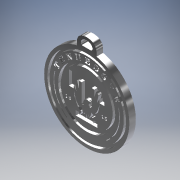
# Autodesk Inventor part: Aluminum Backing
Saved by Autodesk Inventor 2018 (Build 220112000, 112)
## iProperties
Created: 2017-11-28
Part Number: Aluminum Backing
Material: Aluminum 6061
Document SubType Name: Modeling
Designer: Rus
Density: 2.7 g/cm^3
Appearance: Aluminum - Flat
Author: Rus
Autodesk Inventor part; units mm, degrees
(part 1 of 2)
ref_plane "YZ Plane" through (0, 0, 0) normal (1, 0, 0) x (0, 1, 0)
ref_plane "XZ Plane" through (0, 0, 0) normal (0, 1, 0) x (-1, 0, 0)
ref_plane "XY Plane" through (0, 0, 0) normal (0, 0, 1) x (1, 0, 0)
sketch "Sketch1" plane through (0, 0, 0) normal (0, 0, 1) x (1, 0, 0)
  circle A0 centre (0, 0) radius 41.275
  line L0 (-9.525, 40.1609) -> (-9.525, 43.3359)
  line L1 (9.525, 43.3359) -> (9.525, 40.1609)
  line L2 (-9.525, 43.3359) -> (-9.525, 52.8609) construction
  line L3 (-9.525, 52.8609) -> (0, 52.8609) construction
  line L4 (0, 52.8609) -> (9.525, 52.8609) construction
  line L5 (9.525, 52.8609) -> (9.525, 43.3359) construction
  spline S0 degree 4 poles (-9.525, 43.3359) (-9.525, 52.8609) (0, 52.8609) (9.525, 52.8609) (9.525, 43.3359) knots 1 1 1 1 1 2 2 2 2 2
  line L6 (0, 0) -> (0, 52.8609) construction
  line L7 (-9.525, 40.1609) -> (-9.525, 52.8609) construction
  line L8 (-3.7012, 44.5588) -> (3.7012, 44.5588) construction
  line L9 (3.7012, 42.545) -> (-3.7012, 42.545)
  arc A1 (-5.715, 44.5588) -> (-3.7012, 42.545) centre (-3.7012, 44.5588) ccw
  arc A2 (3.7012, 42.545) -> (5.715, 44.5588) centre (3.7012, 44.5588) ccw
  line L10 (-5.715, 44.5588) -> (-5.715, 48.3682) construction
  line L11 (-5.715, 48.3682) -> (0, 51.6703) construction
  line L12 (0, 51.6703) -> (5.715, 48.3682) construction
  line L13 (5.715, 48.3682) -> (5.715, 44.5588) construction
  spline S1 degree 4 poles (-5.715, 44.5588) (-5.715, 48.3682) (0, 51.6703) (5.715, 48.3682) (5.715, 44.5588) knots 0 0 0 0 0 1 1 1 1 1
  point P0 (0, 44.5588)
  point P1 (0, 41.275)
  point P2 (0, 49.1303)
  dimension "d0" = 82.55
  dimension "d1" = 9.525
  dimension "d2" = 12.7
  dimension "d3" = 1.27
  dimension "d4" = 19.05
  dimension "d5" = 3.81
  dimension "d6" = 2.54
  constraints: 14 end point, 7 point on circle, 5 equal length, 5 vertical, 4 point on line, 3 centre point, 3 coincident, 3 horizontal, 2 tangent, 1 collinear, 1 midpoint, 1 parallel, 1 perpendicular, 10 other
  measures "d0" diameter of A0
  measures "d1" distance of L0.end L2.end
  measures "d2" distance of L2.end L0.start
  measures "d3" distance from line of L9 point (0, 41.275)
  measures "d4" distance between parallel lines of L5 L7
  measures "d5" distance from line of L2 L10.start
  measures "d6" distance of L11.end point (0, 49.13)
extrude "Extrusion1" add sketch "Sketch1" against normal blind 6.35
sketch "Sketch2" plane through (0, 0, 0) normal (0, 0, 1) x (1, 0, 0)
  line L0 (-17.3416, 16.1127) -> (17.1721, 16.1127) projected
  line L1 (-17.3416, 2.4226) -> (-17.3416, 16.1127) projected
  line L2 (-12.5842, 2.4226) -> (-17.3416, 2.4226) projected
  line L3 (-12.5842, 2.8144) -> (-12.5842, 2.4226) projected
  line L4 (-12.5284, 3.9883) -> (-12.5842, 2.8144) projected
  line L5 (-12.3951, 5.1768) -> (-12.5284, 3.9883) projected
  line L6 (-12.3568, 5.3992) -> (-12.3951, 5.1768) projected
  line L7 (-10.0045, 1.3116) -> (-12.3568, 5.3992) projected
  line L8 (-11.6489, 8.1267) -> (-10.0045, 1.3116) projected
  line L9 (-11.523, 8.419) -> (-11.6489, 8.1267) projected
  line L10 (-10.7114, 9.6284) -> (-11.523, 8.419) projected
  line L11 (-9.6469, 10.5162) -> (-10.7114, 9.6284) projected
  line L12 (-9.3949, 10.6484) -> (-9.6469, 10.5162) projected
  line L13 (-7.5644, 4.9816) -> (-9.3949, 10.6484) projected
  line L14 (-7.4901, 11.2654) -> (-7.5644, 4.9816) projected
  line L15 (-7.3021, 11.2986) -> (-7.4901, 11.2654) projected
  line L16 (-6.2911, 11.3978) -> (-7.3021, 11.2986) projected
  line L17 (-5.1831, 11.4155) -> (-6.2911, 11.3978) projected
  line L18 (-4.9463, 11.4069) -> (-5.1831, 11.4155) projected
  line L19 (-4.9566, -5.366) -> (-4.9463, 11.4069) projected
  line L20 (-4.9566, -5.5437) -> (-4.9566, -5.366) projected
  line L21 (-4.8688, -6.0783) -> (-4.9566, -5.5437) projected
  line L22 (-4.6042, -6.6704) -> (-4.8688, -6.0783) projected
  line L23 (-4.1619, -7.031) -> (-4.6042, -6.6704) projected
  line L24 (-3.6867, -7.0879) -> (-4.1619, -7.031) projected
  line L25 (-3.5431, -7.0506) -> (-3.6867, -7.0879) projected
  line L26 (-3.4581, -7.0279) -> (-3.5431, -7.0506) projected
  line L27 (-3.2038, -6.7852) -> (-3.4581, -7.0279) projected
  line L28 (-3.1821, -6.3109) -> (-3.2038, -6.7852) projected
  line L29 (-3.2134, -6.1722) -> (-3.1821, -6.3109) projected
  line L30 (-3.2876, -5.8436) -> (-3.2134, -6.1722) projected
  line L31 (-3.3446, -4.8204) -> (-3.2876, -5.8436) projected
  line L32 (-3.148, -3.5625) -> (-3.3446, -4.8204) projected
  line L33 (-2.6706, -2.4546) -> (-3.148, -3.5625) projected
  line L34 (-1.9595, -1.5554) -> (-2.6706, -2.4546) projected
  line L35 (-1.0615, -0.9207) -> (-1.9595, -1.5554) projected
  line L36 (-0.0227, -0.6088) -> (-1.0615, -0.9207) projected
  line L37 (1.1099, -0.6761) -> (-0.0227, -0.6088) projected
  line L38 (2.0206, -1.0117) -> (1.1099, -0.6761) projected
  line L39 (2.2892, -1.1792) -> (2.0206, -1.0117) projected
  line L40 (2.462, -1.1853) -> (2.2892, -1.1792) projected
  line L41 (2.9787, -1.2796) -> (2.462, -1.1853) projected
  line L42 (3.4976, -1.5627) -> (2.9787, -1.2796) projected
  line L43 (3.7921, -2.0846) -> (3.4976, -1.5627) projected
  line L44 (3.8374, -2.7026) -> (3.7921, -2.0846) projected
  line L45 (3.8094, -2.9032) -> (3.8374, -2.7026) projected
  line L46 (3.3827, -2.6573) -> (3.8094, -2.9032) projected
  line L47 (2.5963, -2.8059) -> (3.3827, -2.6573) projected
  line L48 (2.4277, -2.9343) -> (2.5963, -2.8059) projected
  line L49 (2.0515, -3.4873) -> (2.4277, -2.9343) projected
  line L50 (1.9037, -4.2725) -> (2.0515, -3.4873) projected
  line L51 (2.0982, -5.0136) -> (1.9037, -4.2725) projected
  line L52 (2.4329, -5.4662) -> (2.0982, -5.0136) projected
  line L53 (2.5798, -5.5645) -> (2.4329, -5.4662) projected
  line L54 (2.7369, -5.6689) -> (2.5798, -5.5645) projected
  line L55 (3.3322, -5.8013) -> (2.7369, -5.6689) projected
  line L56 (4.0224, -5.5719) -> (3.3322, -5.8013) projected
  line L57 (4.5289, -4.9538) -> (4.0224, -5.5719) projected
  line L58 (4.7252, -4.2592) -> (4.5289, -4.9538) projected
  line L59 (4.7252, -4.0289) -> (4.7252, -4.2592) projected
  line L60 (4.7149, 11.4069) -> (4.7252, -4.0289) projected
  line L61 (4.9505, 11.4155) -> (4.7149, 11.4069) projected
  line L62 (6.0585, 11.3978) -> (4.9505, 11.4155) projected
  line L63 (7.0704, 11.2995) -> (6.0585, 11.3978) projected
  line L64 (7.2586, 11.2666) -> (7.0704, 11.2995) projected
  line L65 (7.3329, 4.9816) -> (7.2586, 11.2666) projected
  line L66 (9.1632, 10.6484) -> (7.3329, 4.9816) projected
  line L67 (9.4155, 10.5162) -> (9.1632, 10.6484) projected
  line L68 (10.4798, 9.6284) -> (9.4155, 10.5162) projected
  line L69 (11.2925, 8.4201) -> (10.4798, 9.6284) projected
  line L70 (11.4184, 8.1277) -> (11.2925, 8.4201) projected
  line L71 (9.7732, 1.3116) -> (11.4184, 8.1277) projected
  line L72 (12.1377, 5.4186) -> (9.7732, 1.3116) projected
  line L73 (12.175, 5.1957) -> (12.1377, 5.4186) projected
  line L74 (12.3063, 3.9997) -> (12.175, 5.1957) projected
  line L75 (12.3633, 2.8173) -> (12.3063, 3.9997) projected
  line L76 (12.3633, 2.4226) -> (12.3633, 2.8173) projected
  line L77 (17.1721, 2.4226) -> (12.3633, 2.4226) projected
  line L78 (17.1721, 16.1127) -> (17.1721, 2.4226) projected
  line L79 (2.2407, -15.384) -> (1.4356, -12.0529) projected
  line L80 (2.1269, -15.5143) -> (2.2407, -15.384) projected
  line L81 (1.5349, -16.0249) -> (2.1269, -15.5143) projected
  line L82 (0.9115, -16.3567) -> (1.5349, -16.0249) projected
  line L83 (0.7833, -16.399) -> (0.9115, -16.3567) projected
  line L84 (-0.0278, -12.3673) -> (0.7833, -16.399) projected
  line L85 (-0.7586, -16.4651) -> (-0.0278, -12.3673) projected
  line L86 (-0.9001, -16.4331) -> (-0.7586, -16.4651) projected
  line L87 (-1.5844, -16.1344) -> (-0.9001, -16.4331) projected
  line L88 (-2.2344, -15.6353) -> (-1.5844, -16.1344) projected
  line L89 (-2.3574, -15.5029) -> (-2.2344, -15.6353) projected
  line L90 (-1.5234, -12.0529) -> (-2.3574, -15.5029) projected
  line L91 (-3.1295, -14.4178) -> (-1.5234, -12.0529) projected
  line L92 (-3.2276, -14.241) -> (-3.1295, -14.4178) projected
  line L93 (-3.6814, -13.2064) -> (-3.2276, -14.241) projected
  line L94 (-4.0826, -11.9569) -> (-3.6814, -13.2064) projected
  line L95 (-4.1537, -11.6736) -> (-4.0826, -11.9569) projected
  line L96 (-4.9589, -9.0011) -> (-4.1537, -11.6736) projected
  line L97 (-5.0075, -9.1787) -> (-4.9589, -9.0011) projected
  line L98 (-5.2597, -9.6833) -> (-5.0075, -9.1787) projected
  line L99 (-5.67, -10.0624) -> (-5.2597, -9.6833) projected
  line L100 (-6.1547, -10.1876) -> (-5.67, -10.0624) projected
  line L101 (-6.6785, -10.11) -> (-6.1547, -10.1876) projected
  line L102 (-7.2057, -9.8774) -> (-6.6785, -10.11) projected
  line L103 (-7.7029, -9.5406) -> (-7.2057, -9.8774) projected
  line L104 (-8.1328, -9.1499) -> (-7.7029, -9.5406) projected
  line L105 (-8.387, -8.8583) -> (-8.1328, -9.1499) projected
  line L106 (-8.4595, -8.754) -> (-8.387, -8.8583) projected
  line L107 (-8.9215, -8.0882) -> (-8.4595, -8.754) projected
  line L108 (-10.1171, -5.9602) -> (-8.9215, -8.0882) projected
  line L109 (-11.3266, -3.1398) -> (-10.1171, -5.9602) projected
  line L110 (-12.1027, -0.4743) -> (-11.3266, -3.1398) projected
  line L111 (-12.4168, 1.2691) -> (-12.1027, -0.4743) projected
  line L112 (-12.4591, 1.8541) -> (-12.4168, 1.2691) projected
  line L113 (-12.4654, 1.7457) -> (-12.4591, 1.8541) projected
  line L114 (-12.4901, 0.5995) -> (-12.4654, 1.7457) projected
  line L115 (-12.4892, 0.4787) -> (-12.4901, 0.5995) projected
  line L116 (-12.4871, -0.1156) -> (-12.4892, 0.4787) projected
  line L117 (-12.2411, -1.9016) -> (-12.4871, -0.1156) projected
  line L118 (-11.499, -4.7419) -> (-12.2411, -1.9016) projected
  line L119 (-10.2455, -7.8052) -> (-11.499, -4.7419) projected
  line L120 (-8.9617, -10.1317) -> (-10.2455, -7.8052) projected
  line L121 (-8.4595, -10.856) -> (-8.9617, -10.1317) projected
  line L122 (-8.3923, -10.9532) -> (-8.4595, -10.856) projected
  line L123 (-8.1772, -11.2366) -> (-8.3923, -10.9532) projected
  line L124 (-7.8021, -11.6914) -> (-8.1772, -11.2366) projected
  line L125 (-7.3586, -12.1678) -> (-7.8021, -11.6914) projected
  line L126 (-6.875, -12.6141) -> (-7.3586, -12.1678) projected
  line L127 (-6.3777, -12.9822) -> (-6.875, -12.6141) projected
  line L128 (-5.8924, -13.2178) -> (-6.3777, -12.9822) projected
  line L129 (-5.4435, -13.2725) -> (-5.8924, -13.2178) projected
  line L130 (-5.1345, -13.162) -> (-5.4435, -13.2725) projected
  line L131 (-5.0601, -13.0948) -> (-5.1345, -13.162) projected
  line L132 (-5.0715, -13.1744) -> (-5.0601, -13.0948) projected
  line L133 (-5.3464, -13.9556) -> (-5.0715, -13.1744) projected
  line L134 (-5.3837, -14.0301) -> (-5.3464, -13.9556) projected
  line L135 (-6.9908, -17.1772) -> (-5.3837, -14.0301) projected
  line L136 (-6.9908, -14.5934) -> (-6.9908, -17.1772) projected
  line L137 (-7.0517, -14.6028) -> (-6.9908, -14.5934) projected
  line L138 (-7.7059, -14.6855) -> (-7.0517, -14.6028) projected
  line L139 (-7.7753, -14.6927) -> (-7.7059, -14.6855) projected
  line L140 (-7.9759, -14.7123) -> (-7.7753, -14.6927) projected
  line L141 (-9.0897, -14.7794) -> (-7.9759, -14.7123) projected
  line L142 (-10.2443, -14.8074) -> (-9.0897, -14.7794) projected
  line L143 (-10.6288, -14.8074) -> (-10.2443, -14.8074) projected
  line L144 (-10.6288, -19.3528) -> (-10.6288, -14.8074) projected
  line L145 (10.4076, -19.3528) -> (-10.6288, -19.3528) projected
  line L146 (10.4076, -14.8074) -> (10.4076, -19.3528) projected
  line L147 (10.015, -14.798) -> (10.4076, -14.8074) projected
  line L148 (8.4108, -14.7401) -> (10.015, -14.798) projected
  line L149 (7.2843, -14.6658) -> (8.4108, -14.7401) projected
  line L150 (7.1302, -14.6481) -> (7.2843, -14.6658) projected
  line L151 (7.1015, -14.6451) -> (7.1302, -14.6481) projected
  line L152 (6.8296, -14.6131) -> (7.1015, -14.6451) projected
  line L153 (6.8037, -14.61) -> (6.8296, -14.6131) projected
  line L154 (6.8037, -17.1772) -> (6.8037, -14.61) projected
  line L155 (5.1448, -13.9278) -> (6.8037, -17.1772) projected
  line L156 (5.1107, -13.8617) -> (5.1448, -13.9278) projected
  line L157 (4.9103, -13.2272) -> (5.1107, -13.8617) projected
  line L158 (4.9, -13.1517) -> (4.9103, -13.2272) projected
  line L159 (4.9783, -13.2076) -> (4.9, -13.1517) projected
  line L160 (5.2875, -13.2788) -> (4.9783, -13.2076) projected
  line L161 (5.732, -13.1931) -> (5.2875, -13.2788) projected
  line L162 (6.2084, -12.9418) -> (5.732, -13.1931) projected
  line L163 (6.6932, -12.5728) -> (6.2084, -12.9418) projected
  line L164 (7.1622, -12.1316) -> (6.6932, -12.5728) projected
  line L165 (7.5903, -11.6676) -> (7.1622, -12.1316) projected
  line L166 (7.9541, -11.2264) -> (7.5903, -11.6676) projected
  line L167 (8.1629, -10.9503) -> (7.9541, -11.2264) projected
  line L168 (8.229, -10.856) -> (8.1629, -10.9503) projected
  line L169 (8.7312, -10.1317) -> (8.229, -10.856) projected
  line L170 (10.014, -7.8052) -> (8.7312, -10.1317) projected
  line L171 (11.2675, -4.7419) -> (10.014, -7.8052) projected
  line L172 (12.0085, -1.9016) -> (11.2675, -4.7419) projected
  line L173 (12.2554, -0.1156) -> (12.0085, -1.9016) projected
  line L174 (12.2575, 0.4787) -> (12.2554, -0.1156) projected
  line L175 (12.2575, 0.5995) -> (12.2575, 0.4787) projected
  line L176 (12.2337, 1.7457) -> (12.2575, 0.5995) projected
  line L177 (12.2288, 1.8541) -> (12.2337, 1.7457) projected
  line L178 (12.1865, 1.2691) -> (12.2288, 1.8541) projected
  line L179 (11.871, -0.4743) -> (12.1865, 1.2691) projected
  line L180 (11.0951, -3.1398) -> (11.871, -0.4743) projected
  line L181 (9.8856, -5.9602) -> (11.0951, -3.1398) projected
  line L182 (8.69, -8.0882) -> (9.8856, -5.9602) projected
  line L183 (8.229, -8.754) -> (8.69, -8.0882) projected
  line L184 (8.1555, -8.8583) -> (8.229, -8.754) projected
  line L185 (7.9002, -9.1499) -> (8.1555, -8.8583) projected
  line L186 (7.4703, -9.5406) -> (7.9002, -9.1499) projected
  line L187 (6.9742, -9.8774) -> (7.4703, -9.5406) projected
  line L188 (6.4461, -10.11) -> (6.9742, -9.8774) projected
  line L189 (5.9221, -10.1876) -> (6.4461, -10.11) projected
  line L190 (5.4374, -10.0624) -> (5.9221, -10.1876) projected
  line L191 (5.0281, -9.6833) -> (5.4374, -10.0624) projected
  line L192 (4.777, -9.1775) -> (5.0281, -9.6833) projected
  line L193 (4.7284, -9.0011) -> (4.777, -9.1775) projected
  line L194 (3.9232, -11.6736) -> (4.7284, -9.0011) projected
  line L195 (3.855, -11.9424) -> (3.9232, -11.6736) projected
  line L196 (3.478, -13.134) -> (3.855, -11.9424) projected
  line L197 (3.0541, -14.1315) -> (3.478, -13.134) projected
  line L198 (2.963, -14.3041) -> (3.0541, -14.1315) projected
  line L199 (1.4356, -12.0529) -> (2.963, -14.3041) projected
  line L200 (-15.909, -6.753) -> (-16.0207, -6.4378) projected
  line L201 (-15.909, -6.9639) -> (-15.909, -6.753) projected
  line L202 (-16.0176, -7.2586) -> (-15.909, -6.9639) projected
  line L203 (-16.0393, -7.2841) -> (-16.0176, -7.2586) projected
  line L204 (-16.0611, -7.3102) -> (-16.0393, -7.2841) projected
  line L205 (-16.3039, -7.4392) -> (-16.0611, -7.3102) projected
  line L206 (-16.488, -7.4392) -> (-16.3039, -7.4392) projected
  line L207 (-16.7731, -7.3112) -> (-16.488, -7.4392) projected
  line L208 (-16.7958, -7.2864) -> (-16.7731, -7.3112) projected
  line L209 (-16.8196, -7.2605) -> (-16.7958, -7.2864) projected
  line L210 (-16.9364, -6.9513) -> (-16.8196, -7.2605) projected
  line L211 (-16.9364, -6.7376) -> (-16.9364, -6.9513) projected
  line L212 (-16.828, -6.4296) -> (-16.9364, -6.7376) projected
  line L213 (-16.8051, -6.4048) -> (-16.828, -6.4296) projected
  line L214 (-16.7834, -6.3789) -> (-16.8051, -6.4048) projected
  line L215 (-16.5209, -6.2539) -> (-16.7834, -6.3789) projected
  line L216 (-16.3359, -6.2539) -> (-16.5209, -6.2539) projected
  line L217 (-16.0652, -6.3852) -> (-16.3359, -6.2539) projected
  line L218 (-16.0424, -6.4118) -> (-16.0652, -6.3852) projected
  line L219 (-16.0207, -6.4378) -> (-16.0424, -6.4118) projected
  line L220 (-16.9231, -8.574) -> (-16.9406, -8.5815) projected
  line L221 (-16.7876, -8.4853) -> (-16.9231, -8.574) projected
  line L222 (-16.7783, -8.4748) -> (-16.7876, -8.4853) projected
  line L223 (-16.7701, -8.4635) -> (-16.7783, -8.4748) projected
  line L224 (-16.7255, -8.35) -> (-16.7701, -8.4635) projected
  line L225 (-16.7255, -8.2559) -> (-16.7255, -8.35) projected
  line L226 (-16.8072, -8.1008) -> (-16.7255, -8.2559) projected
  line L227 (-16.8227, -8.0862) -> (-16.8072, -8.1008) projected
  line L228 (-16.8392, -8.0719) -> (-16.8227, -8.0862) projected
  line L229 (-17.0118, -7.9983) -> (-16.8392, -8.0719) projected
  line L230 (-17.1421, -7.9983) -> (-17.0118, -7.9983) projected
  line L231 (-17.3458, -8.0833) -> (-17.1421, -7.9983) projected
  line L232 (-17.3643, -8.1008) -> (-17.3458, -8.0833) projected
  line L233 (-17.3829, -8.1174) -> (-17.3643, -8.1008) projected
  line L234 (-17.477, -8.3003) -> (-17.3829, -8.1174) projected
  line L235 (-17.477, -8.4689) -> (-17.477, -8.3003) projected
  line L236 (-17.258, -8.7758) -> (-17.477, -8.4689) projected
  line L237 (-17.2134, -8.8057) -> (-17.258, -8.7758) projected
  line L238 (-17.17, -8.8346) -> (-17.2134, -8.8057) projected
  line L239 (-16.7131, -8.9834) -> (-17.17, -8.8346) projected
  line L240 (-16.4, -8.9834) -> (-16.7131, -8.9834) projected
  line L241 (-15.9618, -8.8771) -> (-16.4, -8.9834) projected
  line L242 (-15.5804, -8.6289) -> (-15.9618, -8.8771) projected
  line L243 (-15.5174, -8.5588) -> (-15.5804, -8.6289) projected
  line L244 (-15.4555, -8.4873) -> (-15.5174, -8.5588) projected
  line L245 (-15.2383, -8.0532) -> (-15.4555, -8.4873) projected
  line L246 (-15.1444, -7.5569) -> (-15.2383, -8.0532) projected
  line L247 (-15.1444, -7.2337) -> (-15.1444, -7.5569) projected
  line L248 (-15.2291, -6.7614) -> (-15.1444, -7.2337) projected
  line L249 (-15.4244, -6.356) -> (-15.2291, -6.7614) projected
  line L250 (-15.4802, -6.2911) -> (-15.4244, -6.356) projected
  line L251 (-15.537, -6.2259) -> (-15.4802, -6.2911) projected
  line L252 (-15.8864, -5.9975) -> (-15.537, -6.2259) projected
  line L253 (-16.2946, -5.9005) -> (-15.8864, -5.9975) projected
  line L254 (-16.6388, -5.9005) -> (-16.2946, -5.9005) projected
  line L255 (-17.265, -6.133) -> (-16.6388, -5.9005) projected
  line L256 (-17.3199, -6.1794) -> (-17.265, -6.133) projected
  line L257 (-17.3757, -6.2259) -> (-17.3199, -6.1794) projected
  line L258 (-17.6536, -6.7365) -> (-17.3757, -6.2259) projected
  line L259 (-17.6536, -7.0765) -> (-17.6536, -6.7365) projected
  line L260 (-17.4107, -7.5385) -> (-17.6536, -7.0765) projected
  line L261 (-17.3622, -7.583) -> (-17.4107, -7.5385) projected
  line L262 (-17.3147, -7.6274) -> (-17.3622, -7.583) projected
  line L263 (-16.8175, -7.8507) -> (-17.3147, -7.6274) projected
  line L264 (-16.5447, -7.8507) -> (-16.8175, -7.8507) projected
  line L265 (-16.2687, -7.7937) -> (-16.5447, -7.8507) projected
  line L266 (-16.2378, -7.7825) -> (-16.2687, -7.7937) projected
  line L267 (-16.2068, -7.7711) -> (-16.2378, -7.7825) projected
  line L268 (-15.9008, -7.6015) -> (-16.2068, -7.7711) projected
  line L269 (-15.8709, -7.579) -> (-15.9008, -7.6015) projected
  line L270 (-15.8719, -7.673) -> (-15.8709, -7.579) projected
  line L271 (-16.0197, -8.3746) -> (-15.8719, -7.673) projected
  line L272 (-16.0475, -8.4201) -> (-16.0197, -8.3746) projected
  line L273 (-16.0765, -8.4645) -> (-16.0475, -8.4201) projected
  line L274 (-16.4413, -8.6921) -> (-16.0765, -8.4645) projected
  line L275 (-16.6171, -8.6921) -> (-16.4413, -8.6921) projected
  line L276 (-16.7493, -8.6683) -> (-16.6171, -8.6921) projected
  line L277 (-16.7638, -8.6641) -> (-16.7493, -8.6683) projected
  line L278 (-16.7794, -8.659) -> (-16.7638, -8.6641) projected
  line L279 (-16.9261, -8.5908) -> (-16.7794, -8.659) projected
  line L280 (-16.9406, -8.5815) -> (-16.9261, -8.5908) projected
  line L281 (-18.6728, -8.8923) -> (-20.4701, -8.8923) projected
  line L282 (-18.6728, -8.5485) -> (-18.6728, -8.8923) projected
  line L283 (-18.986, -8.5485) -> (-18.6728, -8.5485) projected
  line L284 (-19.1895, -8.5079) -> (-18.986, -8.5485) projected
  line L285 (-19.1978, -8.5009) -> (-19.1895, -8.5079) projected
  line L286 (-19.2071, -8.4927) -> (-19.1978, -8.5009) projected
  line L287 (-19.2515, -8.3311) -> (-19.2071, -8.4927) projected
  line L288 (-19.2515, -5.9531) -> (-19.2515, -8.3311) projected
  line L289 (-19.6391, -5.9531) -> (-19.2515, -5.9531) projected
  line L290 (-19.6567, -5.9905) -> (-19.6391, -5.9531) projected
  line L291 (-19.9016, -6.2621) -> (-19.6567, -5.9905) projected
  line L292 (-19.9337, -6.2796) -> (-19.9016, -6.2621) projected
  line L293 (-19.9657, -6.2962) -> (-19.9337, -6.2796) projected
  line L294 (-20.4132, -6.3945) -> (-19.9657, -6.2962) projected
  line L295 (-20.4701, -6.3976) -> (-20.4132, -6.3945) projected
  line L296 (-20.4701, -6.7365) -> (-20.4701, -6.3976) projected
  line L297 (-19.882, -6.7365) -> (-20.4701, -6.7365) projected
  line L298 (-19.882, -8.3208) -> (-19.882, -6.7365) projected
  line L299 (-19.9368, -8.4862) -> (-19.882, -8.3208) projected
  line L300 (-19.9471, -8.4955) -> (-19.9368, -8.4862) projected
  line L301 (-19.9585, -8.5039) -> (-19.9471, -8.4955) projected
  line L302 (-20.1796, -8.5485) -> (-19.9585, -8.5039) projected
  line L303 (-20.4701, -8.5485) -> (-20.1796, -8.5485) projected
  line L304 (-20.4701, -8.8923) -> (-20.4701, -8.5485) projected
  line L305 (1.267, -25.1613) -> (5.0705, -24.6497) projected
  line L306 (-1.2682, -25.1613) -> (1.267, -25.1613) projected
  line L307 (-5.0715, -24.6497) -> (-1.2682, -25.1613) projected
  line L308 (-9.7949, -23.1831) -> (-5.0715, -24.6497) projected
  line L309 (-14.0684, -20.8638) -> (-9.7949, -23.1831) projected
  line L310 (-17.7921, -17.7912) -> (-14.0684, -20.8638) projected
  line L311 (-20.8649, -14.0684) -> (-17.7921, -17.7912) projected
  line L312 (-23.1841, -9.7938) -> (-20.8649, -14.0684) projected
  line L313 (-24.6507, -5.0715) -> (-23.1841, -9.7938) projected
  line L314 (-25.1613, -1.2682) -> (-24.6507, -5.0715) projected
  line L315 (-25.1613, 1.267) -> (-25.1613, -1.2682) projected
  line L316 (-24.6507, 5.0705) -> (-25.1613, 1.267) projected
  line L317 (-23.1841, 9.7938) -> (-24.6507, 5.0705) projected
  line L318 (-20.8649, 14.0673) -> (-23.1841, 9.7938) projected
  line L319 (-17.7921, 17.7912) -> (-20.8649, 14.0673) projected
  line L320 (-14.0684, 20.8638) -> (-17.7921, 17.7912) projected
  line L321 (-9.7949, 23.1831) -> (-14.0684, 20.8638) projected
  line L322 (-5.0715, 24.6496) -> (-9.7949, 23.1831) projected
  line L323 (-1.2682, 25.1603) -> (-5.0715, 24.6496) projected
  line L324 (1.267, 25.1603) -> (-1.2682, 25.1603) projected
  line L325 (5.0705, 24.6496) -> (1.267, 25.1603) projected
  line L326 (9.7938, 23.1831) -> (5.0705, 24.6496) projected
  line L327 (14.0673, 20.8638) -> (9.7938, 23.1831) projected
  line L328 (17.7912, 17.7912) -> (14.0673, 20.8638) projected
  line L329 (20.8638, 14.0673) -> (17.7912, 17.7912) projected
  line L330 (23.1831, 9.7938) -> (20.8638, 14.0673) projected
  line L331 (24.6496, 5.0705) -> (23.1831, 9.7938) projected
  line L332 (25.1614, 1.267) -> (24.6496, 5.0705) projected
  line L333 (25.1614, -1.2682) -> (25.1614, 1.267) projected
  line L334 (24.6496, -5.0715) -> (25.1614, -1.2682) projected
  line L335 (23.1831, -9.7938) -> (24.6496, -5.0715) projected
  line L336 (20.8638, -14.0684) -> (23.1831, -9.7938) projected
  line L337 (17.7912, -17.7912) -> (20.8638, -14.0684) projected
  line L338 (14.0673, -20.8638) -> (17.7912, -17.7912) projected
  line L339 (9.7938, -23.1831) -> (14.0673, -20.8638) projected
  line L340 (5.0705, -24.6497) -> (9.7938, -23.1831) projected
  line L341 (-2.8226, 27.4547) -> (-0.706, 27.5962) projected
  line L342 (-5.5624, 27.0361) -> (-2.8226, 27.4547) projected
  line L343 (-8.2073, 26.3559) -> (-5.5624, 27.0361) projected
  line L344 (-10.7427, 25.4277) -> (-8.2073, 26.3559) projected
  line L345 (-13.1548, 24.2663) -> (-10.7427, 25.4277) projected
  line L346 (-15.4305, 22.8832) -> (-13.1548, 24.2663) projected
  line L347 (-17.5546, 21.2947) -> (-15.4305, 22.8832) projected
  line L348 (-19.5151, 19.5141) -> (-17.5546, 21.2947) projected
  line L349 (-21.2959, 17.5534) -> (-19.5151, 19.5141) projected
  line L350 (-22.8844, 15.4294) -> (-21.2959, 17.5534) projected
  line L351 (-24.2672, 13.1538) -> (-22.8844, 15.4294) projected
  line L352 (-25.4289, 10.7415) -> (-24.2672, 13.1538) projected
  line L353 (-26.357, 8.2064) -> (-25.4289, 10.7415) projected
  line L354 (-27.0371, 5.5615) -> (-26.357, 8.2064) projected
  line L355 (-27.4557, 2.8215) -> (-27.0371, 5.5615) projected
  line L356 (-27.5973, 0.7048) -> (-27.4557, 2.8215) projected
  line L357 (-27.5973, -0.706) -> (-27.5973, 0.7048) projected
  line L358 (-27.4557, -2.8215) -> (-27.5973, -0.706) projected
  line L359 (-27.0371, -5.5624) -> (-27.4557, -2.8215) projected
  line L360 (-26.357, -8.2064) -> (-27.0371, -5.5624) projected
  line L361 (-25.4289, -10.7427) -> (-26.357, -8.2064) projected
  line L362 (-24.2672, -13.1548) -> (-25.4289, -10.7427) projected
  line L363 (-22.8844, -15.4295) -> (-24.2672, -13.1548) projected
  line L364 (-21.2959, -17.5546) -> (-22.8844, -15.4295) projected
  line L365 (-19.5151, -19.5141) -> (-21.2959, -17.5546) projected
  line L366 (-17.5546, -21.2948) -> (-19.5151, -19.5141) projected
  line L367 (-15.4305, -22.8834) -> (-17.5546, -21.2948) projected
  line L368 (-13.1548, -24.2662) -> (-15.4305, -22.8834) projected
  line L369 (-10.7427, -25.4279) -> (-13.1548, -24.2662) projected
  line L370 (-8.2073, -26.356) -> (-10.7427, -25.4279) projected
  line L371 (-5.5624, -27.0361) -> (-8.2073, -26.356) projected
  line L372 (-2.8226, -27.4547) -> (-5.5624, -27.0361) projected
  line L373 (-0.706, -27.5973) -> (-2.8226, -27.4547) projected
  line L374 (0.7048, -27.5973) -> (-0.706, -27.5973) projected
  line L375 (2.8215, -27.4547) -> (0.7048, -27.5973) projected
  line L376 (5.5615, -27.0361) -> (2.8215, -27.4547) projected
  line L377 (8.2064, -26.356) -> (5.5615, -27.0361) projected
  line L378 (10.7415, -25.4279) -> (8.2064, -26.356) projected
  line L379 (13.1538, -24.2662) -> (10.7415, -25.4279) projected
  line L380 (15.4294, -22.8834) -> (13.1538, -24.2662) projected
  line L381 (17.5534, -21.2948) -> (15.4294, -22.8834) projected
  line L382 (19.5141, -19.5141) -> (17.5534, -21.2948) projected
  line L383 (21.2947, -17.5546) -> (19.5141, -19.5141) projected
  line L384 (22.8832, -15.4295) -> (21.2947, -17.5546) projected
  line L385 (24.2663, -13.1548) -> (22.8832, -15.4295) projected
  line L386 (25.4277, -10.7427) -> (24.2663, -13.1548) projected
  line L387 (26.3559, -8.2064) -> (25.4277, -10.7427) projected
  line L388 (27.0361, -5.5624) -> (26.3559, -8.2064) projected
  line L389 (27.4547, -2.8215) -> (27.0361, -5.5624) projected
  line L390 (27.5974, -0.706) -> (27.4547, -2.8215) projected
  line L391 (27.5974, 0.7048) -> (27.5974, -0.706) projected
  line L392 (27.4547, 2.8215) -> (27.5974, 0.7048) projected
  line L393 (27.0361, 5.5615) -> (27.4547, 2.8215) projected
  line L394 (26.3559, 8.2064) -> (27.0361, 5.5615) projected
  line L395 (25.4277, 10.7415) -> (26.3559, 8.2064) projected
  line L396 (24.2663, 13.1538) -> (25.4277, 10.7415) projected
  line L397 (22.8832, 15.4294) -> (24.2663, 13.1538) projected
  line L398 (21.2947, 17.5534) -> (22.8832, 15.4294) projected
  line L399 (19.5141, 19.5141) -> (21.2947, 17.5534) projected
  line L400 (17.5534, 21.2947) -> (19.5141, 19.5141) projected
  line L401 (15.4294, 22.8832) -> (17.5534, 21.2947) projected
  line L402 (13.1538, 24.2663) -> (15.4294, 22.8832) projected
  line L403 (10.7415, 25.4277) -> (13.1538, 24.2663) projected
  line L404 (8.2064, 26.3559) -> (10.7415, 25.4277) projected
  line L405 (5.5615, 27.0361) -> (8.2064, 26.3559) projected
  line L406 (2.8215, 27.4547) -> (5.5615, 27.0361) projected
  line L407 (0.7048, 27.5962) -> (2.8215, 27.4547) projected
  line L408 (-0.706, 27.5962) -> (0.7048, 27.5962) projected
  line L409 (-31.1816, 3.914) -> (-31.4255, 0.9776) projected
  line L410 (-30.6266, 7.0716) -> (-31.1816, 3.914) projected
  line L411 (-30.4705, 7.6865) -> (-30.6266, 7.0716) projected
  line L412 (-31.1733, 7.9532) -> (-30.4705, 7.6865) projected
  line L413 (-31.3366, 7.3173) -> (-31.1733, 7.9532) projected
  line L414 (-31.9164, 4.0516) -> (-31.3366, 7.3173) projected
  line L415 (-32.1706, 1.0129) -> (-31.9164, 4.0516) projected
  line L416 (-32.1706, -0.9634) -> (-32.1706, 1.0129) projected
  line L417 (-31.9422, -3.85) -> (-32.1706, -0.9634) projected
  line L418 (-31.2725, -7.5655) -> (-31.9422, -3.85) projected
  line L419 (-30.1883, -11.1206) -> (-31.2725, -7.5655) projected
  line L420 (-28.7156, -14.49) -> (-30.1883, -11.1206) projected
  line L421 (-26.8831, -17.6475) -> (-28.7156, -14.49) projected
  line L422 (-24.7148, -20.5652) -> (-26.8831, -17.6475) projected
  line L423 (-22.2395, -23.2172) -> (-24.7148, -20.5652) projected
  line L424 (-20.2014, -25.029) -> (-22.2395, -23.2172) projected
  line L425 (-19.481, -25.5788) -> (-20.2014, -25.029) projected
  line L426 (-19.0355, -24.9814) -> (-19.481, -25.5788) projected
  line L427 (-19.7394, -24.444) -> (-19.0355, -24.9814) projected
  line L428 (-21.7289, -22.6746) -> (-19.7394, -24.444) projected
  line L429 (-24.1463, -20.0835) -> (-21.7289, -22.6746) projected
  line L430 (-26.263, -17.2342) -> (-24.1463, -20.0835) projected
  line L431 (-28.052, -14.1511) -> (-26.263, -17.2342) projected
  line L432 (-29.4897, -10.8614) -> (-28.052, -14.1511) projected
  line L433 (-30.548, -7.3887) -> (-29.4897, -10.8614) projected
  line L434 (-31.2022, -3.7599) -> (-30.548, -7.3887) projected
  line L435 (-31.4255, -0.9405) -> (-31.2022, -3.7599) projected
  line L436 (-31.4255, 0.9776) -> (-31.4255, -0.9405) projected
  circle A0 centre (0, 0) radius 38.1 projected
  line L437 (0.919, -35.9523) -> (3.6753, -35.7663) projected
  line L438 (-0.9199, -35.9523) -> (0.919, -35.9523) projected
  line L439 (-3.6765, -35.7663) -> (-0.9199, -35.9523) projected
  line L440 (-7.2462, -35.2216) -> (-3.6765, -35.7663) projected
  line L441 (-10.6918, -34.3359) -> (-7.2462, -35.2216) projected
  line L442 (-13.9951, -33.1267) -> (-10.6918, -34.3359) projected
  line L443 (-17.137, -31.6125) -> (-13.9951, -33.1267) projected
  line L444 (-20.1011, -29.8121) -> (-17.137, -31.6125) projected
  line L445 (-22.8689, -27.742) -> (-20.1011, -29.8121) projected
  line L446 (-25.4217, -25.4217) -> (-22.8689, -27.742) projected
  line L447 (-27.743, -22.8689) -> (-25.4217, -25.4217) projected
  line L448 (-29.8121, -20.1011) -> (-27.743, -22.8689) projected
  line L449 (-31.6125, -17.137) -> (-29.8121, -20.1011) projected
  line L450 (-33.1267, -13.9939) -> (-31.6125, -17.137) projected
  line L451 (-34.3359, -10.6907) -> (-33.1267, -13.9939) projected
  line L452 (-35.2216, -7.2462) -> (-34.3359, -10.6907) projected
  line L453 (-35.7663, -3.6765) -> (-35.2216, -7.2462) projected
  line L454 (-35.9513, -0.9199) -> (-35.7663, -3.6765) projected
  line L455 (-35.9513, 0.919) -> (-35.9513, -0.9199) projected
  line L456 (-35.7663, 3.6753) -> (-35.9513, 0.919) projected
  line L457 (-35.2216, 7.2451) -> (-35.7663, 3.6753) projected
  line L458 (-34.3359, 10.6897) -> (-35.2216, 7.2451) projected
  line L459 (-33.1267, 13.993) -> (-34.3359, 10.6897) projected
  line L460 (-31.6125, 17.136) -> (-33.1267, 13.993) projected
  line L461 (-29.8121, 20.1) -> (-31.6125, 17.136) projected
  line L462 (-27.743, 22.868) -> (-29.8121, 20.1) projected
  line L463 (-25.4217, 25.4207) -> (-27.743, 22.868) projected
  line L464 (-22.8689, 27.741) -> (-25.4217, 25.4207) projected
  line L465 (-20.1011, 29.8112) -> (-22.8689, 27.741) projected
  line L466 (-17.137, 31.6116) -> (-20.1011, 29.8112) projected
  line L467 (-13.9951, 33.1257) -> (-17.137, 31.6116) projected
  line L468 (-10.6918, 34.335) -> (-13.9951, 33.1257) projected
  line L469 (-7.2462, 35.2206) -> (-10.6918, 34.335) projected
  line L470 (-3.6765, 35.7652) -> (-7.2462, 35.2206) projected
  line L471 (-0.9199, 35.9502) -> (-3.6765, 35.7652) projected
  line L472 (0.919, 35.9502) -> (-0.9199, 35.9502) projected
  line L473 (3.6753, 35.7652) -> (0.919, 35.9502) projected
  line L474 (7.2451, 35.2206) -> (3.6753, 35.7652) projected
  line L475 (10.6907, 34.335) -> (7.2451, 35.2206) projected
  line L476 (13.9941, 33.1257) -> (10.6907, 34.335) projected
  line L477 (17.137, 31.6116) -> (13.9941, 33.1257) projected
  line L478 (20.1012, 29.8112) -> (17.137, 31.6116) projected
  line L479 (22.869, 27.741) -> (20.1012, 29.8112) projected
  line L480 (25.4217, 25.4207) -> (22.869, 27.741) projected
  line L481 (27.7421, 22.868) -> (25.4217, 25.4207) projected
  line L482 (29.8121, 20.1) -> (27.7421, 22.868) projected
  line L483 (31.6123, 17.136) -> (29.8121, 20.1) projected
  line L484 (33.1266, 13.993) -> (31.6123, 17.136) projected
  line L485 (34.3357, 10.6897) -> (33.1266, 13.993) projected
  line L486 (35.2215, 7.2451) -> (34.3357, 10.6897) projected
  line L487 (35.7664, 3.6753) -> (35.2215, 7.2451) projected
  line L488 (35.9523, 0.919) -> (35.7664, 3.6753) projected
  line L489 (35.9523, -0.9199) -> (35.9523, 0.919) projected
  line L490 (35.7664, -3.6765) -> (35.9523, -0.9199) projected
  line L491 (35.2215, -7.2462) -> (35.7664, -3.6765) projected
  line L492 (34.3357, -10.6907) -> (35.2215, -7.2462) projected
  line L493 (33.1266, -13.9939) -> (34.3357, -10.6907) projected
  line L494 (31.6123, -17.137) -> (33.1266, -13.9939) projected
  line L495 (29.8121, -20.1011) -> (31.6123, -17.137) projected
  line L496 (27.7421, -22.8689) -> (29.8121, -20.1011) projected
  line L497 (25.4217, -25.4217) -> (27.7421, -22.8689) projected
  line L498 (22.869, -27.742) -> (25.4217, -25.4217) projected
  line L499 (20.1012, -29.8121) -> (22.869, -27.742) projected
  line L500 (17.137, -31.6125) -> (20.1012, -29.8121) projected
  line L501 (13.9941, -33.1267) -> (17.137, -31.6125) projected
  line L502 (10.6907, -34.3359) -> (13.9941, -33.1267) projected
  line L503 (7.2451, -35.2216) -> (10.6907, -34.3359) projected
  line L504 (3.6753, -35.7663) -> (7.2451, -35.2216) projected
  line L505 (17.7613, -8.4418) -> (17.6929, -8.4418) projected
  line L506 (17.9668, -8.3614) -> (17.7613, -8.4418) projected
  line L507 (17.9857, -8.3458) -> (17.9668, -8.3614) projected
  line L508 (18.003, -8.329) -> (17.9857, -8.3458) projected
  line L509 (18.0941, -8.1505) -> (18.003, -8.329) projected
  line L510 (18.0941, -8.0263) -> (18.0941, -8.1505) projected
  line L511 (18.0021, -7.8518) -> (18.0941, -8.0263) projected
  line L512 (17.9834, -7.8362) -> (18.0021, -7.8518) projected
  line L513 (17.9647, -7.8198) -> (17.9834, -7.8362) projected
  line L514 (17.7695, -7.7402) -> (17.9647, -7.8198) projected
  line L515 (17.6258, -7.7402) -> (17.7695, -7.7402) projected
  line L516 (17.4109, -7.8436) -> (17.6258, -7.7402) projected
  line L517 (17.3911, -7.8642) -> (17.4109, -7.8436) projected
  line L518 (17.3704, -7.8848) -> (17.3911, -7.8642) projected
  line L519 (17.2673, -8.0936) -> (17.3704, -7.8848) projected
  line L520 (17.2673, -8.3056) -> (17.2673, -8.0936) projected
  line L521 (17.5452, -8.7106) -> (17.2673, -8.3056) projected
  line L522 (17.6009, -8.7487) -> (17.5452, -8.7106) projected
  line L523 (17.6557, -8.7861) -> (17.6009, -8.7487) projected
  line L524 (18.2531, -8.9741) -> (17.6557, -8.7861) projected
  line L525 (18.6016, -8.9741) -> (18.2531, -8.9741) projected
  line L526 (18.9921, -8.8977) -> (18.6016, -8.9741) projected
  line L527 (19.3331, -8.722) -> (18.9921, -8.8977) projected
  line L528 (19.3889, -8.6723) -> (19.3331, -8.722) projected
  line L529 (19.4447, -8.6216) -> (19.3889, -8.6723) projected
  line L530 (19.64, -8.3159) -> (19.4447, -8.6216) projected
  line L531 (19.7238, -7.9675) -> (19.64, -8.3159) projected
  line L532 (19.7238, -7.6783) -> (19.7238, -7.9675) projected
  line L533 (19.448, -7.1601) -> (19.7238, -7.6783) projected
  line L534 (19.3931, -7.1117) -> (19.448, -7.1601) projected
  line L535 (19.3373, -7.062) -> (19.3931, -7.1117) projected
  line L536 (18.7583, -6.8184) -> (19.3373, -7.062) projected
  line L537 (18.4629, -6.8184) -> (18.7583, -6.8184) projected
  line L538 (18.2118, -6.8532) -> (18.4629, -6.8184) projected
  line L539 (18.1819, -6.8607) -> (18.2118, -6.8532) projected
  line L540 (18.151, -6.8677) -> (18.1819, -6.8607) projected
  line L541 (17.843, -6.9752) -> (18.151, -6.8677) projected
  line L542 (17.8117, -6.9898) -> (17.843, -6.9752) projected
  line L543 (17.8491, -6.5517) -> (17.8117, -6.9898) projected
  line L544 (17.8799, -6.5555) -> (17.8491, -6.5517) projected
  line L545 (18.1385, -6.5858) -> (17.8799, -6.5555) projected
  line L546 (18.1592, -6.5877) -> (18.1385, -6.5858) projected
  line L547 (18.1787, -6.5886) -> (18.1592, -6.5877) projected
  line L548 (18.3202, -6.598) -> (18.1787, -6.5886) projected
  line L549 (18.5642, -6.598) -> (18.3202, -6.598) projected
  line L550 (19.1336, -6.4574) -> (18.5642, -6.598) projected
  line L551 (19.1833, -6.4296) -> (19.1336, -6.4574) projected
  line L552 (19.2329, -6.4016) -> (19.1833, -6.4296) projected
  line L553 (19.5596, -5.9727) -> (19.2329, -6.4016) projected
  line L554 (19.576, -5.9148) -> (19.5596, -5.9727) projected
  line L555 (19.5369, -5.9272) -> (19.576, -5.9148) projected
  line L556 (19.1243, -6.0192) -> (19.5369, -5.9272) projected
  line L557 (19.082, -6.0253) -> (19.1243, -6.0192) projected
  line L558 (19.0386, -6.0316) -> (19.082, -6.0253) projected
  line L559 (18.678, -6.0627) -> (19.0386, -6.0316) projected
  line L560 (18.4236, -6.0627) -> (18.678, -6.0627) projected
  line L561 (18.0661, -6.0307) -> (18.4236, -6.0627) projected
  line L562 (18.0259, -6.0246) -> (18.0661, -6.0307) projected
  line L563 (17.9845, -6.0183) -> (18.0259, -6.0246) projected
  line L564 (17.5833, -5.9223) -> (17.9845, -6.0183) projected
  line L565 (17.5443, -5.9097) -> (17.5833, -5.9223) projected
  line L566 (17.3963, -7.4579) -> (17.5443, -5.9097) projected
  line L567 (17.7211, -7.4724) -> (17.3963, -7.4579) projected
  line L568 (17.7428, -7.4457) -> (17.7211, -7.4724) projected
  line L569 (17.9752, -7.2544) -> (17.7428, -7.4457) projected
  line L570 (18, -7.2419) -> (17.9752, -7.2544) projected
  line L571 (18.0247, -7.2283) -> (18, -7.2419) projected
  line L572 (18.2449, -7.1664) -> (18.0247, -7.2283) projected
  line L573 (18.4476, -7.1664) -> (18.2449, -7.1664) projected
  line L574 (18.8071, -7.3308) -> (18.4476, -7.1664) projected
  line L575 (18.8382, -7.364) -> (18.8071, -7.3308) projected
  line L576 (18.8683, -7.396) -> (18.8382, -7.364) projected
  line L577 (19.0212, -7.7774) -> (18.8683, -7.396) projected
  line L578 (19.0212, -8.042) -> (19.0212, -7.7774) projected
  line L579 (18.862, -8.4201) -> (19.0212, -8.042) projected
  line L580 (18.8309, -8.4521) -> (18.862, -8.4201) projected
  line L581 (18.7989, -8.4841) -> (18.8309, -8.4521) projected
  line L582 (18.432, -8.6434) -> (18.7989, -8.4841) projected
  line L583 (18.2242, -8.6434) -> (18.432, -8.6434) projected
  line L584 (17.9977, -8.6022) -> (18.2242, -8.6434) projected
  line L585 (17.9731, -8.5936) -> (17.9977, -8.6022) projected
  line L586 (17.9472, -8.5843) -> (17.9731, -8.5936) projected
  line L587 (17.7136, -8.4584) -> (17.9472, -8.5843) projected
  line L588 (17.6929, -8.4418) -> (17.7136, -8.4584) projected
  line L589 (16.2232, -8.8923) -> (14.4258, -8.8923) projected
  line L590 (16.2232, -8.5485) -> (16.2232, -8.8923) projected
  line L591 (15.9113, -8.5485) -> (16.2232, -8.5485) projected
  line L592 (15.7065, -8.5079) -> (15.9113, -8.5485) projected
  line L593 (15.6983, -8.5009) -> (15.7065, -8.5079) projected
  line L594 (15.689, -8.4927) -> (15.6983, -8.5009) projected
  line L595 (15.6456, -8.3311) -> (15.689, -8.4927) projected
  line L596 (15.6456, -5.9531) -> (15.6456, -8.3311) projected
  line L597 (15.257, -5.9531) -> (15.6456, -5.9531) projected
  line L598 (15.2394, -5.9905) -> (15.257, -5.9531) projected
  line L599 (14.9944, -6.2621) -> (15.2394, -5.9905) projected
  line L600 (14.9636, -6.2796) -> (14.9944, -6.2621) projected
  line L601 (14.9316, -6.2962) -> (14.9636, -6.2796) projected
  line L602 (14.4828, -6.3945) -> (14.9316, -6.2962) projected
  line L603 (14.4258, -6.3976) -> (14.4828, -6.3945) projected
  line L604 (14.4258, -6.7365) -> (14.4258, -6.3976) projected
  line L605 (15.0141, -6.7365) -> (14.4258, -6.7365) projected
  line L606 (15.0141, -8.3208) -> (15.0141, -6.7365) projected
  line L607 (14.9603, -8.4862) -> (15.0141, -8.3208) projected
  line L608 (14.9501, -8.4955) -> (14.9603, -8.4862) projected
  line L609 (14.9386, -8.5039) -> (14.9501, -8.4955) projected
  line L610 (14.7175, -8.5485) -> (14.9386, -8.5039) projected
  line L611 (14.4258, -8.5485) -> (14.7175, -8.5485) projected
  line L612 (14.4258, -8.8923) -> (14.4258, -8.5485) projected
  line L613 (31.9154, 4.0516) -> (32.1707, 1.0129) projected
  line L614 (31.3357, 7.3173) -> (31.9154, 4.0516) projected
  line L615 (31.1732, 7.9532) -> (31.3357, 7.3173) projected
  line L616 (30.4705, 7.6865) -> (31.1732, 7.9532) projected
  line L617 (30.6255, 7.0716) -> (30.4705, 7.6865) projected
  line L618 (31.1807, 3.914) -> (30.6255, 7.0716) projected
  line L619 (31.4255, 0.9776) -> (31.1807, 3.914) projected
  line L620 (31.4255, -0.9405) -> (31.4255, 0.9776) projected
  line L621 (31.2012, -3.7599) -> (31.4255, -0.9405) projected
  line L622 (30.5469, -7.3887) -> (31.2012, -3.7599) projected
  line L623 (29.4886, -10.8614) -> (30.5469, -7.3887) projected
  line L624 (28.0519, -14.1511) -> (29.4886, -10.8614) projected
  line L625 (26.2619, -17.2342) -> (28.0519, -14.1511) projected
  line L626 (24.1453, -20.0835) -> (26.2619, -17.2342) projected
  line L627 (21.7279, -22.6746) -> (24.1453, -20.0835) projected
  line L628 (19.7385, -24.444) -> (21.7279, -22.6746) projected
  line L629 (19.0355, -24.9814) -> (19.7385, -24.444) projected
  line L630 (19.4821, -25.5788) -> (19.0355, -24.9814) projected
  line L631 (20.2014, -25.029) -> (19.4821, -25.5788) projected
  line L632 (22.2384, -23.2172) -> (20.2014, -25.029) projected
  line L633 (24.7147, -20.5652) -> (22.2384, -23.2172) projected
  line L634 (26.8822, -17.6475) -> (24.7147, -20.5652) projected
  line L635 (28.7156, -14.4911) -> (26.8822, -17.6475) projected
  line L636 (30.1874, -11.1218) -> (28.7156, -14.4911) projected
  line L637 (31.2713, -7.5655) -> (30.1874, -11.1218) projected
  line L638 (31.9413, -3.85) -> (31.2713, -7.5655) projected
  line L639 (32.1707, -0.9634) -> (31.9413, -3.85) projected
  line L640 (32.1707, 1.0129) -> (32.1707, -0.9634) projected
  line L641 (25.1521, 15.3625) -> (25.7318, 15.6496) projected
  line L642 (27.3192, 10.9947) -> (25.1521, 15.3625) projected
  line L643 (29.1425, 11.8992) -> (27.3192, 10.9947) projected
  line L644 (28.8552, 12.4777) -> (29.1425, 11.8992) projected
  line L645 (28.7247, 12.4294) -> (28.8552, 12.4777) projected
  line L646 (28.1761, 12.2897) -> (28.7247, 12.4294) projected
  line L647 (27.7606, 12.2928) -> (28.1761, 12.2897) projected
  line L648 (27.6976, 12.3145) -> (27.7606, 12.2928) projected
  line L649 (27.6345, 12.3372) -> (27.6976, 12.3145) projected
  line L650 (27.3236, 12.5955) -> (27.6345, 12.3372) projected
  line L651 (27.0196, 13.0525) -> (27.3236, 12.5955) projected
  line L652 (26.9598, 13.1733) -> (27.0196, 13.0525) projected
  line L653 (26.666, 13.7644) -> (26.9598, 13.1733) projected
  line L654 (28.0904, 14.4713) -> (26.666, 13.7644) projected
  line L655 (28.145, 14.3618) -> (28.0904, 14.4713) projected
  line L656 (28.1761, 14.2989) -> (28.145, 14.3618) projected
  line L657 (28.2639, 13.8316) -> (28.1761, 14.2989) projected
  line L658 (28.2504, 13.8006) -> (28.2639, 13.8316) projected
  line L659 (28.2361, 13.7707) -> (28.2504, 13.8006) projected
  line L660 (27.7884, 13.4222) -> (28.2361, 13.7707) projected
  line L661 (27.713, 13.3821) -> (27.7884, 13.4222) projected
  line L662 (27.9839, 12.8269) -> (27.713, 13.3821) projected
  line L663 (30.0013, 13.8276) -> (27.9839, 12.8269) projected
  line L664 (29.7264, 14.3807) -> (30.0013, 13.8276) projected
  line L665 (29.6561, 14.3466) -> (29.7264, 14.3807) projected
  line L666 (29.1393, 14.2182) -> (29.6561, 14.3466) projected
  line L667 (29.1063, 14.2267) -> (29.1393, 14.2182) projected
  line L668 (29.0722, 14.2359) -> (29.1063, 14.2267) projected
  line L669 (28.7539, 14.5883) -> (29.0722, 14.2359) projected
  line L670 (28.724, 14.6493) -> (28.7539, 14.5883) projected
  line L671 (28.6701, 14.7588) -> (28.724, 14.6493) projected
  line L672 (29.9277, 15.3821) -> (28.6701, 14.7588) projected
  line L673 (30.2112, 14.8095) -> (29.9277, 15.3821) projected
  line L674 (30.2525, 14.7268) -> (30.2112, 14.8095) projected
  line L675 (30.4985, 14.1303) -> (30.2525, 14.7268) projected
  line L676 (30.5067, 14.0943) -> (30.4985, 14.1303) projected
  line L677 (30.5139, 14.0581) -> (30.5067, 14.0943) projected
  line L678 (30.5078, 13.7274) -> (30.5139, 14.0581) projected
  line L679 (30.4985, 13.6975) -> (30.5078, 13.7274) projected
  line L680 (30.489, 13.6684) -> (30.4985, 13.6975) projected
  line L681 (30.3122, 13.376) -> (30.489, 13.6684) projected
  line L682 (30.2855, 13.347) -> (30.3122, 13.376) projected
  line L683 (30.2586, 13.3192) -> (30.2855, 13.347) projected
  line L684 (29.8247, 12.9706) -> (30.2586, 13.3192) projected
  line L685 (29.7656, 12.9294) -> (29.8247, 12.9706) projected
  line L686 (30.0529, 12.3507) -> (29.7656, 12.9294) projected
  line L687 (31.7375, 13.1858) -> (30.0529, 12.3507) projected
  line L688 (29.5715, 17.5546) -> (31.7375, 13.1858) projected
  line L689 (28.9926, 17.2673) -> (29.5715, 17.5546) projected
  line L690 (29.1134, 17.0223) -> (28.9926, 17.2673) projected
  line L691 (29.1341, 16.9798) -> (29.1134, 17.0223) projected
  line L692 (29.2191, 16.679) -> (29.1341, 16.9798) projected
  line L693 (29.2147, 16.6617) -> (29.2191, 16.679) projected
  line L694 (29.2096, 16.6449) -> (29.2147, 16.6617) projected
  line L695 (28.973, 16.4518) -> (29.2096, 16.6449) projected
  line L696 (28.9307, 16.4301) -> (28.973, 16.4518) projected
  line L697 (26.4345, 15.1929) -> (28.9307, 16.4301) projected
  line L698 (26.3923, 15.1722) -> (26.4345, 15.1929) projected
  line L699 (26.0966, 15.1007) -> (26.3923, 15.1722) projected
  line L700 (26.08, 15.1072) -> (26.0966, 15.1007) projected
  line L701 (26.0625, 15.1143) -> (26.08, 15.1072) projected
  line L702 (25.8733, 15.3625) -> (26.0625, 15.1143) projected
  line L703 (25.8528, 15.4048) -> (25.8733, 15.3625) projected
  line L704 (25.7318, 15.6496) -> (25.8528, 15.4048) projected
  line L705 (19.8914, 21.7414) -> (20.3677, 22.1784) projected
  line L706 (23.184, 18.1457) -> (19.8914, 21.7414) projected
  line L707 (24.6859, 19.5202) -> (23.184, 18.1457) projected
  line L708 (24.2486, 19.9977) -> (24.6859, 19.5202) projected
  line L709 (24.1371, 19.9153) -> (24.2486, 19.9977) projected
  line L710 (23.6471, 19.6289) -> (24.1371, 19.9153) projected
  line L711 (23.2482, 19.5162) -> (23.6471, 19.6289) projected
  line L712 (23.1819, 19.519) -> (23.2482, 19.5162) projected
  line L713 (23.1149, 19.5234) -> (23.1819, 19.519) projected
  line L714 (22.7449, 19.6855) -> (23.1149, 19.5234) projected
  line L715 (22.3253, 20.04) -> (22.7449, 19.6855) projected
  line L716 (22.2342, 20.1393) -> (22.3253, 20.04) projected
  line L717 (21.789, 20.6262) -> (22.2342, 20.1393) projected
  line L718 (22.9608, 21.7) -> (21.789, 20.6262) projected
  line L719 (23.0446, 21.6101) -> (22.9608, 21.7) projected
  line L720 (23.092, 21.5583) -> (23.0446, 21.6101) projected
  line L721 (23.305, 21.1346) -> (23.092, 21.5583) projected
  line L722 (23.3008, 21.1015) -> (23.305, 21.1346) projected
  line L723 (23.2957, 21.0685) -> (23.3008, 21.1015) projected
  line L724 (22.9629, 20.6087) -> (23.2957, 21.0685) projected
  line L725 (22.901, 20.5496) -> (22.9629, 20.6087) projected
  line L726 (23.3143, 20.0918) -> (22.901, 20.5496) projected
  line L727 (24.9753, 21.6122) -> (23.3143, 20.0918) projected
  line L728 (24.5587, 22.0679) -> (24.9753, 21.6122) projected
  line L729 (24.501, 22.0151) -> (24.5587, 22.0679) projected
  line L730 (24.0379, 21.7484) -> (24.501, 22.0151) projected
  line L731 (24.0038, 21.7475) -> (24.0379, 21.7484) projected
  line L732 (23.9685, 21.7475) -> (24.0038, 21.7475) projected
  line L733 (23.5654, 21.9978) -> (23.9685, 21.7475) projected
  line L734 (23.5201, 22.0471) -> (23.5654, 21.9978) projected
  line L735 (23.4384, 22.1372) -> (23.5201, 22.0471) projected
  line L736 (24.4739, 23.085) -> (23.4384, 22.1372) projected
  line L737 (24.905, 22.6137) -> (24.4739, 23.085) projected
  line L738 (24.9669, 22.5455) -> (24.905, 22.6137) projected
  line L739 (25.3691, 22.041) -> (24.9669, 22.5455) projected
  line L740 (25.3866, 22.0081) -> (25.3691, 22.041) projected
  line L741 (25.4043, 21.9761) -> (25.3866, 22.0081) projected
  line L742 (25.49, 21.6566) -> (25.4043, 21.9761) projected
  line L743 (25.49, 21.6244) -> (25.49, 21.6566) projected
  line L744 (25.4889, 21.5945) -> (25.49, 21.6244) projected
  line L745 (25.399, 21.2648) -> (25.4889, 21.5945) projected
  line L746 (25.3815, 21.2297) -> (25.399, 21.2648) projected
  line L747 (25.3626, 21.1945) -> (25.3815, 21.2297) projected
  line L748 (25.0433, 20.7399) -> (25.3626, 21.1945) projected
  line L749 (24.9978, 20.683) -> (25.0433, 20.7399) projected
  line L750 (25.434, 20.2065) -> (24.9978, 20.683) projected
  line L751 (26.8222, 21.4768) -> (25.434, 20.2065) projected
  line L752 (23.5294, 25.0725) -> (26.8222, 21.4768) projected
  line L753 (23.0528, 24.6362) -> (23.5294, 25.0725) projected
  line L754 (23.2368, 24.4356) -> (23.0528, 24.6362) projected
  line L755 (23.2688, 24.4008) -> (23.2368, 24.4356) projected
  line L756 (23.4323, 24.135) -> (23.2688, 24.4008) projected
  line L757 (23.433, 24.1162) -> (23.4323, 24.135) projected
  line L758 (23.433, 24.0988) -> (23.433, 24.1162) projected
  line L759 (23.2595, 23.8487) -> (23.433, 24.0988) projected
  line L760 (23.2242, 23.8157) -> (23.2595, 23.8487) projected
  line L761 (21.1708, 21.9346) -> (23.2242, 23.8157) projected
  line L762 (21.1358, 21.9025) -> (21.1708, 21.9346) projected
  line L763 (20.8712, 21.7526) -> (21.1358, 21.9025) projected
  line L764 (20.8535, 21.7549) -> (20.8712, 21.7526) projected
  line L765 (20.8348, 21.7566) -> (20.8535, 21.7549) projected
  line L766 (20.5837, 21.942) -> (20.8348, 21.7566) projected
  line L767 (20.5517, 21.977) -> (20.5837, 21.942) projected
  line L768 (20.3677, 22.1784) -> (20.5517, 21.977) projected
  line L769 (14.2079, 25.6636) -> (13.7025, 25.9796) projected
  line L770 (14.5656, 25.863) -> (14.2079, 25.6636) projected
  line L771 (14.5873, 25.8103) -> (14.5656, 25.863) projected
  line L772 (14.9468, 25.2677) -> (14.5873, 25.8103) projected
  line L773 (14.9977, 25.2129) -> (14.9468, 25.2677) projected
  line L774 (15.0472, 25.1582) -> (14.9977, 25.2129) projected
  line L775 (15.6147, 24.6848) -> (15.0472, 25.1582) projected
  line L776 (15.6787, 24.6446) -> (15.6147, 24.6848) projected
  line L777 (15.8109, 24.5617) -> (15.6787, 24.6446) projected
  line L778 (16.4508, 24.2889) -> (15.8109, 24.5617) projected
  line L779 (17.0574, 24.2084) -> (16.4508, 24.2889) projected
  line L780 (17.1741, 24.2207) -> (17.0574, 24.2084) projected
  line L781 (17.29, 24.2343) -> (17.1741, 24.2207) projected
  line L782 (17.7942, 24.4337) -> (17.29, 24.2343) projected
  line L783 (18.1973, 24.8161) -> (17.7942, 24.4337) projected
  line L784 (18.2623, 24.9195) -> (18.1973, 24.8161) projected
  line L785 (18.3171, 25.0085) -> (18.2623, 24.9195) projected
  line L786 (18.4878, 25.8983) -> (18.3171, 25.0085) projected
  line L787 (18.4671, 25.9871) -> (18.4878, 25.8983) projected
  line L788 (18.4454, 26.0772) -> (18.4671, 25.9871) projected
  line L789 (18.2188, 26.5462) -> (18.4454, 26.0772) projected
  line L790 (17.8323, 27.0455) -> (18.2188, 26.5462) projected
  line L791 (17.7314, 27.1497) -> (17.8323, 27.0455) projected
  line L792 (17.7055, 27.1767) -> (17.7314, 27.1497) projected
  line L793 (17.3509, 27.5301) -> (17.7055, 27.1767) projected
  line L794 (17.3064, 27.5735) -> (17.3509, 27.5301) projected
  line L795 (17.1865, 27.6892) -> (17.3064, 27.5735) projected
  line L796 (16.8185, 28.1709) -> (17.1865, 27.6892) projected
  line L797 (16.7566, 28.5295) -> (16.8185, 28.1709) projected
  line L798 (16.7907, 28.582) -> (16.7566, 28.5295) projected
  line L799 (16.8135, 28.6194) -> (16.7907, 28.582) projected
  line L800 (17.1492, 28.82) -> (16.8135, 28.6194) projected
  line L801 (17.1938, 28.8221) -> (17.1492, 28.82) projected
  line L802 (17.237, 28.8251) -> (17.1938, 28.8221) projected
  line L803 (17.7199, 28.6752) -> (17.237, 28.8251) projected
  line L804 (17.7725, 28.6422) -> (17.7199, 28.6752) projected
  line L805 (17.8594, 28.5874) -> (17.7725, 28.6422) projected
  line L806 (18.432, 27.9227) -> (17.8594, 28.5874) projected
  line L807 (18.46, 27.8442) -> (18.432, 27.9227) projected
  line L808 (18.4867, 27.7667) -> (18.46, 27.8442) projected
  line L809 (18.4269, 26.9617) -> (18.4867, 27.7667) projected
  line L810 (18.3874, 26.879) -> (18.4269, 26.9617) projected
  line L811 (18.9601, 26.5203) -> (18.3874, 26.879) projected
  line L812 (19.917, 28.0479) -> (18.9601, 26.5203) projected
  line L813 (19.3992, 28.3723) -> (19.917, 28.0479) projected
  line L814 (19.0902, 28.1544) -> (19.3992, 28.3723) projected
  line L815 (19.0706, 28.2081) -> (19.0902, 28.1544) projected
  line L816 (18.7566, 28.7104) -> (19.0706, 28.2081) projected
  line L817 (18.714, 28.7571) -> (18.7566, 28.7104) projected
  line L818 (18.6705, 28.8044) -> (18.714, 28.7571) projected
  line L819 (18.1186, 29.2499) -> (18.6705, 28.8044) projected
  line L820 (18.0518, 29.2922) -> (18.1186, 29.2499) projected
  line L821 (17.9163, 29.377) -> (18.0518, 29.2922) projected
  line L822 (17.2764, 29.6572) -> (17.9163, 29.377) projected
  line L823 (16.6855, 29.743) -> (17.2764, 29.6572) projected
  line L824 (16.5748, 29.7304) -> (16.6855, 29.743) projected
  line L825 (16.4632, 29.7191) -> (16.5748, 29.7304) projected
  line L826 (15.9763, 29.5195) -> (16.4632, 29.7191) projected
  line L827 (15.5795, 29.132) -> (15.9763, 29.5195) projected
  line L828 (15.5134, 29.0267) -> (15.5795, 29.132) projected
  line L829 (15.4842, 28.9811) -> (15.5134, 29.0267) projected
  line L830 (15.3107, 28.5036) -> (15.4842, 28.9811) projected
  line L831 (15.3055, 28.454) -> (15.3107, 28.5036) projected
  line L832 (15.2992, 28.4055) -> (15.3055, 28.454) projected
  line L833 (15.3593, 27.9124) -> (15.2992, 28.4055) projected
  line L834 (15.3768, 27.8631) -> (15.3593, 27.9124) projected
  line L835 (15.3903, 27.8237) -> (15.3768, 27.8631) projected
  line L836 (15.6157, 27.4143) -> (15.3903, 27.8237) projected
  line L837 (15.6477, 27.3708) -> (15.6157, 27.4143) projected
  line L838 (15.6787, 27.3286) -> (15.6477, 27.3708) projected
  line L839 (15.9277, 27.0373) -> (15.6787, 27.3286) projected
  line L840 (16.2996, 26.6422) -> (15.9277, 27.0373) projected
  line L841 (16.3927, 26.5483) -> (16.2996, 26.6422) projected
  line L842 (16.5343, 26.4067) -> (16.3927, 26.5483) projected
  line L843 (16.5522, 26.389) -> (16.5343, 26.4067) projected
  line L844 (16.6585, 26.2827) -> (16.5522, 26.389) projected
  line L845 (16.9747, 25.8175) -> (16.6585, 26.2827) projected
  line L846 (17.0027, 25.4455) -> (16.9747, 25.8175) projected
  line L847 (16.9654, 25.3843) -> (17.0027, 25.4455) projected
  line L848 (16.9404, 25.3462) -> (16.9654, 25.3843) projected
  line L849 (16.583, 25.1479) -> (16.9404, 25.3462) projected
  line L850 (16.5354, 25.1458) -> (16.583, 25.1479) projected
  line L851 (16.4878, 25.1447) -> (16.5354, 25.1458) projected
  line L852 (15.9569, 25.3224) -> (16.4878, 25.1447) projected
  line L853 (15.8978, 25.3588) -> (15.9569, 25.3224) projected
  line L854 (15.8121, 25.4125) -> (15.8978, 25.3588) projected
  line L855 (15.4711, 25.7306) -> (15.8121, 25.4125) projected
  line L856 (15.2455, 26.1153) -> (15.4711, 25.7306) projected
  line L857 (15.2189, 26.2019) -> (15.2455, 26.1153) projected
  line L858 (15.1909, 26.2888) -> (15.2189, 26.2019) projected
  line L859 (15.252, 27.1807) -> (15.1909, 26.2888) projected
  line L860 (15.2922, 27.2716) -> (15.252, 27.1807) projected
  line L861 (14.7319, 27.6231) -> (15.2922, 27.2716) projected
  line L862 (13.7025, 25.9796) -> (14.7319, 27.6231) projected
  line L863 (7.0723, 28.4704) -> (6.502, 28.6443) projected
  line L864 (7.3661, 28.756) -> (7.0723, 28.4704) projected
  line L865 (7.4011, 28.7104) -> (7.3661, 28.756) projected
  line L866 (7.8888, 28.2816) -> (7.4011, 28.7104) projected
  line L867 (7.952, 28.2411) -> (7.8888, 28.2816) projected
  line L868 (8.014, 28.202) -> (7.952, 28.2411) projected
  line L869 (8.6857, 27.8928) -> (8.014, 28.202) projected
  line L870 (8.7582, 27.8702) -> (8.6857, 27.8928) projected
  line L871 (8.908, 27.8246) -> (8.7582, 27.8702) projected
  line L872 (9.5964, 27.7275) -> (8.908, 27.8246) projected
  line L873 (10.202, 27.8071) -> (9.5964, 27.7275) projected
  line L874 (10.3116, 27.8496) -> (10.202, 27.8071) projected
  line L875 (10.4202, 27.8919) -> (10.3116, 27.8496) projected
  line L876 (10.8562, 28.2172) -> (10.4202, 27.8919) projected
  line L877 (11.1444, 28.6916) -> (10.8562, 28.2172) projected
  line L878 (11.1808, 28.8086) -> (11.1444, 28.6916) projected
  line L879 (11.2107, 28.9089) -> (11.1808, 28.8086) projected
  line L880 (11.2509, 29.378) -> (11.2107, 28.9089) projected
  line L881 (11.1435, 29.8112) -> (11.2509, 29.378) projected
  line L882 (11.1001, 29.8917) -> (11.1435, 29.8112) projected
  line L883 (11.0557, 29.9733) -> (11.1001, 29.8917) projected
  line L884 (10.2123, 30.7496) -> (11.0557, 29.9733) projected
  line L885 (10.0883, 30.824) -> (10.2123, 30.7496) projected
  line L886 (10.0563, 30.8435) -> (10.0883, 30.824) projected
  line L887 (9.621, 31.0917) -> (10.0563, 30.8435) projected
  line L888 (9.5663, 31.1216) -> (9.621, 31.0917) projected
  line L889 (9.4204, 31.2024) -> (9.5663, 31.1216) projected
  line L890 (8.94, 31.5712) -> (9.4204, 31.2024) projected